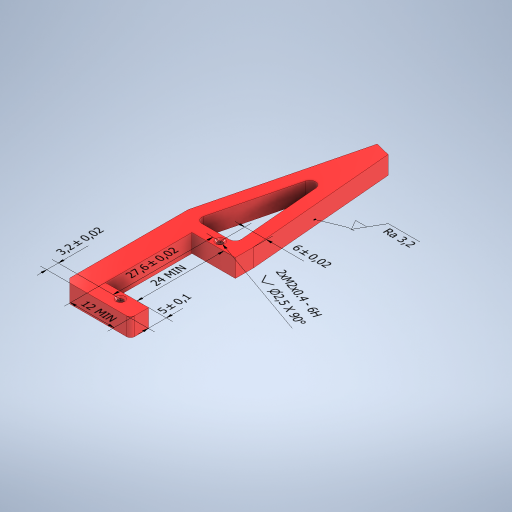
# Autodesk Inventor part: rapoukLegv9
Saved by Autodesk Inventor 2024 (Build 280153000, 153)
## iProperties
Created: 2023-06-22
Part Number: rapoukLegv9
Material: EN AW-6060 T6
Document SubType Name: Modeling
Designer: Roman
Density: 2.7 g/cm^3
Appearance: Light Red
Mass: 15.4015 g
Surface Area: 41.4189 cm^2
Volume: 5.70428 cm^3
Description: Přední noha
Polotovar: KR...
Author: Roman
## iProperties of the stored document MemberDocs/xIbcejt23Mcnw1njhJ3dlasc4Ob
Created: 2023-06-22
Part Number: rapoukLegv9
Material: EN AW-6060 T6
Document SubType Name: Modeling
Designer: Roman
Density: 2.7 g/cm^3
Appearance: Light Red
Mass: 15.4015 g
Surface Area: 41.4189 cm^2
Volume: 5.70428 cm^3
Description: Přední noha
Polotovar: KR...
Author: Roman
## iProperties of the stored document rapoukLegv9_3DPrint.ipt
Created: 2024-08-16
Part Number: rapoukLegv9_3DPrint
Material: Generic
Document SubType Name: Modeling
Designer: Roman Suk
Density: 1 g/cm^3
Appearance: Default
Author: Roman Suk
Autodesk Inventor part; units mm, degrees
ref_plane "YZ Plane" through (0, 0, 0) normal (1, 0, 0) x (0, 1, 0)
ref_plane "XZ Plane" through (0, 0, 0) normal (0, 1, 0) x (-1, 0, 0)
ref_plane "XY Plane" through (0, 0, 0) normal (0, 0, 1) x (1, 0, 0)
sketch "Sketch1" plane through (0, 0, 0) normal (0, 1, 0) x (-1, 0, 0)
  line L0 (0, 0) -> (18, 0)
  line L1 (0, 0) -> (0, -5)
  line L2 (0, -5) -> (3.5719, -45.8274)
  line L3 (18, 0) -> (18, -5)
  line L4 (18, -5) -> (7.5719, -46.8247)
  line L5 (3.5719, -45.8274) -> (7.5719, -46.8247)
  dimension "d0" = 18
  dimension "d1" = 5
  dimension "d3" = 175
  dimension "d6" = 76
  dimension "d7" = 4
  constraints: 12 end point, 2 vertical, 1 horizontal, 1 parallel, 1 perpendicular
  measures "d0" distance of L0.start L0.end
  measures "d1" distance of L0.start L1.end
  measures "d3" angle of L2 L1
  measures "d6" angle of L0 L4
  measures "d7" horizontal distance of L4.end L2.end
extrude "Extrusion1" add sketch "Sketch1" along normal blind 5
shell "Shell1" thickness 3.5 removed faces 2 at (-7.1906, 5, -18.6091) at (-7.1906, 0, -18.6091)
fillet "Fillet1" radius 1.5875 5 edges at (-14.5, 2.5, -3.5) (-3.5, 2.5, -3.5) (-14.5, 2.5, -4.5703) (-6.3393, 2.5, -37.3009) (-3.5, 2.5, -4.8472)
sketch "Sketch2" plane through (0, 0, 0) normal (0, -1, 0) x (1, 0, 0)
  line L0 (0, 0) -> (-12, 0)
  line L1 (-12, 0) -> (-12, 24)
  line L2 (-12, 24) -> (0, 24)
  line L3 (0, 24) -> (0, 0)
  line L4 (0, 24) -> (-12, 24)
  line L5 (-12, 24) -> (-12, 29)
  line L6 (-12, 29) -> (0, 29)
  line L7 (0, 29) -> (0, 24)
  line L8 (-12, 0) -> (-18, 0)
  line L9 (-18, 0) -> (-18, 24)
  line L10 (-18, 24) -> (-12, 24)
  line L11 (-12, 24) -> (-12, 0)
  line L12 (-18, 24) -> (-13.7574, 24) construction
  line L13 (-12, 29) -> (-16.8, 29)
  line L14 (-16.8, 29) -> (-18, 27.8)
  line L15 (-18, 27.8) -> (-18, 24)
  dimension "d14" = 24
  dimension "d15" = 5
  dimension "d16" = 12
  dimension "d18" = 6
  dimension "d57" = 1.2
  dimension "d58" = 135
  constraints: 32 end point, 6 parallel, 5 horizontal, 4 perpendicular, 2 collinear
  measures "d14" distance of L0.end L1.end
  measures "d15" distance of L4.end L5.end
  measures "d16" distance between parallel lines of L7 L5
  measures "d18" distance between parallel lines of L9 L1
  measures "d57" horizontal distance of L14.end L13.end
  measures "d58" angle of L13 L14
extrude "Extrusion2" add sketch "Sketch2" against normal blind 5 contours L8 L9 L10 L1 | L2 L5 L6 L7 | L10 L15 L14 L13 L5
fillet "Fillet3" radius 1 1 edges at (0, 2.5, 29)
sketch "Sketch4" plane through (0, 5, 0) normal (0, 1, 0) x (1, 0, 0)
  line L0 (-12, -24) -> (-12, 0) projected
  line L1 (-12, -12) -> (-18, -12)
  line L2 (-18, 5) -> (-18, -29) projected
  line L3 (0, -24) -> (-12, -24) projected
  line L4 (-12, 0) -> (0, 0) projected
  circle A0 centre (-6, -25.8) radius 0.8
  circle A1 centre (-6, 1.8) radius 0.8
  line L5 (0, -28) -> (0, -24) projected
  point P0 (-18, 1.9304)
  point P1 (-18, -27.8)
  point P2 (-16.8, -29)
  dimension "d31" = 1.6
  dimension "d32" = 27.6
  dimension "d43" = 6
  dimension "d46" = 13.8
  constraints: 2 centre point, 2 end point, 1 horizontal, 1 midpoint, 1 symmetric about line, 3 other
  measures "d31" diameter of A0
  measures "d32" distance of A1.centre A0.centre
  measures "d43" horizontal distance of L0.start A0.centre
  measures "d46" vertical distance of A0.centre L1.end
hole "Hole1" at (-6, 5, 25.8) at (-6, 5, -1.8) direction (0, -1, 0) diameter 1.567 depth 10 countersink diameter 2.5 countersink angle 90 thread size "M2x0.4" class "6H" standard "ISO Metric profile"
body "Solid1"
